9 th pillar (Autodesk Fusion 360 design; units mm, degrees)
description: Spur Gear; Module: 1.27; Num Teeth: 9; Pressure Angle: 20.0; Backlash: 0.00 mm
part number: 2026-06-06-19-48-23-059
Autodesk Fusion 360 part; units mm, degrees
sketch "Base Circle" plane through (0, 0, 0) normal (0, 0, 1) x (1, 0, 0)
  circle A0 centre (0, 0) radius 4.2456
  circle A1 centre (0, 0) radius 2.5
extrude "Extrude1" add sketch "Base Circle" along normal blind 1
sketch "Gear Tooth" plane through (0, 0, 0) normal (0, 0, 1) x (1, 0, 0)
  spline S0 degree 5 poles (5.2743, -1.0113) (5.279, -1.0122) (5.2884, -1.0138) (5.3026, -1.0158) (5.3217, -1.0174) (5.3456, -1.0181) (5.3698, -1.0179) (5.394, -1.0171) (5.4182, -1.016) (5.4425, -1.0146) (5.4668, -1.013) (5.4912, -1.0111) (5.5156, -1.0088) (5.5401, -1.0061) (5.5646, -1.0028) (5.5892, -0.9991) (5.6137, -0.995) (5.6383, -0.9906) (5.663, -0.9859) (5.6876, -0.981) (5.7122, -0.9757) (5.7369, -0.9702) (5.7616, -0.9644) (5.7863, -0.9583) (5.811, -0.9518) (5.8357, -0.9451) (5.8604, -0.9381) (5.8851, -0.9308) (5.9098, -0.9233) (5.9345, -0.9155) (5.9592, -0.9074) (5.9839, -0.8991) (6.0086, -0.8905) (6.0333, -0.8817) (6.058, -0.8726) (6.0827, -0.8632) (6.1073, -0.8537) (6.132, -0.8438) (6.1566, -0.8338) (6.1812, -0.8234) (6.2058, -0.8129) (6.2304, -0.8021) (6.255, -0.7911) (6.2795, -0.7799) (6.304, -0.7684) (6.3285, -0.7567) (6.353, -0.7448) (6.3774, -0.7326) (6.4018, -0.7203) (6.4262, -0.7077) (6.4505, -0.6948) (6.4748, -0.6818) (6.4991, -0.6686) (6.5233, -0.6551) (6.5475, -0.6414) (6.5717, -0.6275) (6.5958, -0.6134) (6.6199, -0.5991) (6.644, -0.5846) (6.668, -0.5698) (6.6919, -0.5549) (6.7159, -0.5397) (6.7397, -0.5244) (6.7636, -0.5088) (6.7874, -0.493) (6.8111, -0.4771) (6.8348, -0.4609) (6.8584, -0.4445) (6.882, -0.4279) (6.9055, -0.4112) (6.929, -0.3942) (6.9477, -0.3805) (6.9617, -0.3701) (6.9711, -0.3631) (6.9757, -0.3597) knots 0 0 0 0 0 0 0.01428571 0.02857143 0.04285714 0.05714286 0.07142857 0.08571429 0.1 0.11428571 0.12857143 0.14285714 0.15714286 0.17142857 0.18571429 0.2 0.21428571 0.22857143 0.24285714 0.25714286 0.27142857 0.28571429 0.3 0.31428571 0.32857143 0.34285714 0.35714286 0.37142857 0.38571429 0.4 0.41428571 0.42857143 0.44285714 0.45714286 0.47142857 0.48571429 0.5 0.51428571 0.52857143 0.54285714 0.55714286 0.57142857 0.58571429 0.6 0.61428571 0.62857143 0.64285714 0.65714286 0.67142857 0.68571429 0.7 0.71428571 0.72857143 0.74285714 0.75714286 0.77142857 0.78571429 0.8 0.81428571 0.82857143 0.84285714 0.85714286 0.87142857 0.88571429 0.9 0.91428571 0.92857143 0.94285714 0.95714286 0.97142857 0.98571429 1 1 1 1 1 1
  spline S1 degree 5 poles (5.2743, 1.0113) (5.279, 1.0122) (5.2884, 1.0138) (5.3026, 1.0158) (5.3217, 1.0174) (5.3456, 1.0181) (5.3698, 1.0179) (5.394, 1.0171) (5.4182, 1.016) (5.4425, 1.0146) (5.4668, 1.013) (5.4912, 1.0111) (5.5156, 1.0088) (5.5401, 1.0061) (5.5646, 1.0028) (5.5892, 0.9991) (5.6137, 0.995) (5.6383, 0.9906) (5.663, 0.9859) (5.6876, 0.981) (5.7122, 0.9757) (5.7369, 0.9702) (5.7616, 0.9644) (5.7863, 0.9583) (5.811, 0.9518) (5.8357, 0.9451) (5.8604, 0.9381) (5.8851, 0.9308) (5.9098, 0.9233) (5.9345, 0.9155) (5.9592, 0.9074) (5.9839, 0.8991) (6.0086, 0.8905) (6.0333, 0.8817) (6.058, 0.8726) (6.0827, 0.8632) (6.1073, 0.8537) (6.132, 0.8438) (6.1566, 0.8338) (6.1812, 0.8234) (6.2058, 0.8129) (6.2304, 0.8021) (6.255, 0.7911) (6.2795, 0.7799) (6.304, 0.7684) (6.3285, 0.7567) (6.353, 0.7448) (6.3774, 0.7326) (6.4018, 0.7203) (6.4262, 0.7077) (6.4505, 0.6948) (6.4748, 0.6818) (6.4991, 0.6686) (6.5233, 0.6551) (6.5475, 0.6414) (6.5717, 0.6275) (6.5958, 0.6134) (6.6199, 0.5991) (6.644, 0.5846) (6.668, 0.5698) (6.6919, 0.5549) (6.7159, 0.5397) (6.7397, 0.5244) (6.7636, 0.5088) (6.7874, 0.493) (6.8111, 0.4771) (6.8348, 0.4609) (6.8584, 0.4445) (6.882, 0.4279) (6.9055, 0.4112) (6.929, 0.3942) (6.9477, 0.3805) (6.9617, 0.3701) (6.9711, 0.3631) (6.9757, 0.3597) knots 0 0 0 0 0 0 0.01428571 0.02857143 0.04285714 0.05714286 0.07142857 0.08571429 0.1 0.11428571 0.12857143 0.14285714 0.15714286 0.17142857 0.18571429 0.2 0.21428571 0.22857143 0.24285714 0.25714286 0.27142857 0.28571429 0.3 0.31428571 0.32857143 0.34285714 0.35714286 0.37142857 0.38571429 0.4 0.41428571 0.42857143 0.44285714 0.45714286 0.47142857 0.48571429 0.5 0.51428571 0.52857143 0.54285714 0.55714286 0.57142857 0.58571429 0.6 0.61428571 0.62857143 0.64285714 0.65714286 0.67142857 0.68571429 0.7 0.71428571 0.72857143 0.74285714 0.75714286 0.77142857 0.78571429 0.8 0.81428571 0.82857143 0.84285714 0.85714286 0.87142857 0.88571429 0.9 0.91428571 0.92857143 0.94285714 0.95714286 0.97142857 0.98571429 1 1 1 1 1 1
  arc A0 (6.9757, -0.3597) -> (6.9757, 0.3597) centre (0, 0) ccw
  line L0 (4.1598, -0.7976) -> (5.2743, -1.0113)
  line L1 (4.1598, 0.7976) -> (5.2743, 1.0113)
  line L2 (4.1598, -0.7976) -> (4.1598, 0.7976)
  point P0 (5.3906, -1.0171)
  point P1 (5.5093, -1.0094)
  point P2 (5.6296, -0.9922)
  point P3 (5.751, -0.9669)
  point P4 (5.8732, -0.9343)
  point P5 (5.9959, -0.8949)
  point P6 (6.1191, -0.8489)
  point P7 (6.2424, -0.7967)
  point P8 (6.3656, -0.7384)
  point P9 (6.4887, -0.6742)
  point P10 (6.6115, -0.6041)
  point P11 (6.7336, -0.5282)
  point P12 (6.8551, -0.4467)
  point P13 (5.3906, 1.0171)
  point P14 (5.5093, 1.0094)
  point P15 (5.6296, 0.9922)
  point P16 (5.751, 0.9669)
  point P17 (5.8732, 0.9343)
  point P18 (5.9959, 0.8949)
  point P19 (6.1191, 0.8489)
  point P20 (6.2424, 0.7967)
  point P21 (6.3656, 0.7384)
  point P22 (6.4887, 0.6742)
  point P23 (6.6115, 0.6041)
  point P24 (6.7336, 0.5282)
  point P25 (6.8551, 0.4467)
extrude "Extrude2" add sketch "Gear Tooth" along normal blind 1
fillet "Fillet1" radius 0.2 2 edges at (4.1697, -0.7995, 0.5) (4.1697, 0.7995, 0.5)
pattern_circular "C-Pattern1" count 9 over 360 about axis through (0, 0, 0) along (0, 0, 1) of "Extrude2", "Fillet1"
sketch "Diametrial Pitch Circle" plane through (0, 0, 0) normal (0, 0, 1) x (1, 0, 0)
  circle A0 centre (0, 0) radius 5.715 construction
extrude "Extrude3" add 1 faces at (-1.8218, -3.1555, 1) along direction (0, 0, 1) blind 23
sketch "Sketch4" plane through (0, 0, 24) normal (0, 0, 1) x (1, 0, 0)
  arc A0 (3.7973, -1.8989) -> (4.1295, -0.9863) centre (0, 0) ccw
  arc A1 (4.3617, -0.8363) -> (4.1295, -0.9863) centre (4.324, -1.0327) ccw
  line L0 (4.3617, -0.8363) -> (5.2743, -1.0113)
  spline S0 degree 5 poles (5.2743, -1.0113) (5.279, -1.0122) (5.2884, -1.0138) (5.3026, -1.0158) (5.3217, -1.0174) (5.3456, -1.0181) (5.3698, -1.0179) (5.394, -1.0171) (5.4182, -1.016) (5.4425, -1.0146) (5.4668, -1.013) (5.4912, -1.0111) (5.5156, -1.0088) (5.5401, -1.0061) (5.5646, -1.0028) (5.5892, -0.9991) (5.6137, -0.995) (5.6383, -0.9906) (5.663, -0.9859) (5.6876, -0.981) (5.7122, -0.9757) (5.7369, -0.9702) (5.7616, -0.9644) (5.7863, -0.9583) (5.811, -0.9518) (5.8357, -0.9451) (5.8604, -0.9381) (5.8851, -0.9308) (5.9098, -0.9233) (5.9345, -0.9155) (5.9592, -0.9074) (5.9839, -0.8991) (6.0086, -0.8905) (6.0333, -0.8817) (6.058, -0.8726) (6.0827, -0.8632) (6.1073, -0.8537) (6.132, -0.8438) (6.1566, -0.8338) (6.1812, -0.8234) (6.2058, -0.8129) (6.2304, -0.8021) (6.255, -0.7911) (6.2795, -0.7799) (6.304, -0.7684) (6.3285, -0.7567) (6.353, -0.7448) (6.3774, -0.7326) (6.4018, -0.7203) (6.4262, -0.7077) (6.4505, -0.6948) (6.4748, -0.6818) (6.4991, -0.6686) (6.5233, -0.6551) (6.5475, -0.6414) (6.5717, -0.6275) (6.5958, -0.6134) (6.6199, -0.5991) (6.644, -0.5846) (6.668, -0.5698) (6.6919, -0.5549) (6.7159, -0.5397) (6.7397, -0.5244) (6.7636, -0.5088) (6.7874, -0.493) (6.8111, -0.4771) (6.8348, -0.4609) (6.8584, -0.4445) (6.882, -0.4279) (6.9055, -0.4112) (6.929, -0.3942) (6.9477, -0.3805) (6.9617, -0.3701) (6.9711, -0.3631) (6.9757, -0.3597) knots 0 0 0 0 0 0 0.01428571 0.02857143 0.04285714 0.05714286 0.07142857 0.08571429 0.1 0.11428571 0.12857143 0.14285714 0.15714286 0.17142857 0.18571429 0.2 0.21428571 0.22857143 0.24285714 0.25714286 0.27142857 0.28571429 0.3 0.31428571 0.32857143 0.34285714 0.35714286 0.37142857 0.38571429 0.4 0.41428571 0.42857143 0.44285714 0.45714286 0.47142857 0.48571429 0.5 0.51428571 0.52857143 0.54285714 0.55714286 0.57142857 0.58571429 0.6 0.61428571 0.62857143 0.64285714 0.65714286 0.67142857 0.68571429 0.7 0.71428571 0.72857143 0.74285714 0.75714286 0.77142857 0.78571429 0.8 0.81428571 0.82857143 0.84285714 0.85714286 0.87142857 0.88571429 0.9 0.91428571 0.92857143 0.94285714 0.95714286 0.97142857 0.98571429 1 1 1 1 1 1
  arc A2 (6.9757, -0.3597) -> (6.9757, 0.3597) centre (0, 0) ccw
  spline S1 degree 5 poles (6.9757, 0.3597) (6.9711, 0.3631) (6.9617, 0.3701) (6.9477, 0.3805) (6.929, 0.3942) (6.9055, 0.4112) (6.882, 0.4279) (6.8584, 0.4445) (6.8348, 0.4609) (6.8111, 0.4771) (6.7874, 0.493) (6.7636, 0.5088) (6.7397, 0.5244) (6.7159, 0.5397) (6.6919, 0.5549) (6.668, 0.5698) (6.644, 0.5846) (6.6199, 0.5991) (6.5958, 0.6134) (6.5717, 0.6275) (6.5475, 0.6414) (6.5233, 0.6551) (6.4991, 0.6686) (6.4748, 0.6818) (6.4505, 0.6948) (6.4262, 0.7077) (6.4018, 0.7203) (6.3774, 0.7326) (6.353, 0.7448) (6.3285, 0.7567) (6.304, 0.7684) (6.2795, 0.7799) (6.255, 0.7911) (6.2304, 0.8021) (6.2058, 0.8129) (6.1812, 0.8234) (6.1566, 0.8338) (6.132, 0.8438) (6.1073, 0.8537) (6.0827, 0.8632) (6.058, 0.8726) (6.0333, 0.8817) (6.0086, 0.8905) (5.9839, 0.8991) (5.9592, 0.9074) (5.9345, 0.9155) (5.9098, 0.9233) (5.8851, 0.9308) (5.8604, 0.9381) (5.8357, 0.9451) (5.811, 0.9518) (5.7863, 0.9583) (5.7616, 0.9644) (5.7369, 0.9702) (5.7122, 0.9757) (5.6876, 0.981) (5.663, 0.9859) (5.6383, 0.9906) (5.6137, 0.995) (5.5892, 0.9991) (5.5646, 1.0028) (5.5401, 1.0061) (5.5156, 1.0088) (5.4912, 1.0111) (5.4668, 1.013) (5.4425, 1.0146) (5.4182, 1.016) (5.394, 1.0171) (5.3698, 1.0179) (5.3456, 1.0181) (5.3217, 1.0174) (5.3026, 1.0158) (5.2884, 1.0138) (5.279, 1.0122) (5.2743, 1.0113) knots -1 -1 -1 -1 -1 -1 -0.98571429 -0.97142857 -0.95714286 -0.94285714 -0.92857143 -0.91428571 -0.9 -0.88571429 -0.87142857 -0.85714286 -0.84285714 -0.82857143 -0.81428571 -0.8 -0.78571429 -0.77142857 -0.75714286 -0.74285714 -0.72857143 -0.71428571 -0.7 -0.68571429 -0.67142857 -0.65714286 -0.64285714 -0.62857143 -0.61428571 -0.6 -0.58571429 -0.57142857 -0.55714286 -0.54285714 -0.52857143 -0.51428571 -0.5 -0.48571429 -0.47142857 -0.45714286 -0.44285714 -0.42857143 -0.41428571 -0.4 -0.38571429 -0.37142857 -0.35714286 -0.34285714 -0.32857143 -0.31428571 -0.3 -0.28571429 -0.27142857 -0.25714286 -0.24285714 -0.22857143 -0.21428571 -0.2 -0.18571429 -0.17142857 -0.15714286 -0.14285714 -0.12857143 -0.11428571 -0.1 -0.08571429 -0.07142857 -0.05714286 -0.04285714 -0.02857143 -0.01428571 0 0 0 0 0 0
  line L1 (5.2743, 1.0113) -> (4.3617, 0.8363)
  arc A3 (4.1295, 0.9863) -> (4.3617, 0.8363) centre (4.324, 1.0327) ccw
  arc A4 (4.1295, 0.9863) -> (3.7973, 1.8989) centre (0, 0) ccw
  arc A5 (3.8788, 2.163) -> (3.7973, 1.8989) centre (3.9762, 1.9883) ccw
  line L2 (3.8788, 2.163) -> (4.6904, 2.6156)
  spline S2 degree 5 poles (4.6904, 2.6156) (4.6945, 2.6179) (4.7028, 2.6227) (4.7149, 2.6303) (4.7306, 2.6413) (4.7494, 2.6562) (4.7678, 2.6719) (4.7858, 2.688) (4.8036, 2.7045) (4.8214, 2.7211) (4.839, 2.738) (4.8565, 2.7551) (4.8737, 2.7726) (4.8906, 2.7904) (4.9073, 2.8087) (4.9238, 2.8273) (4.94, 2.8462) (4.956, 2.8654) (4.9718, 2.8848) (4.9875, 2.9044) (5.003, 2.9243) (5.0184, 2.9444) (5.0335, 2.9647) (5.0485, 2.9853) (5.0633, 3.0061) (5.0779, 3.0271) (5.0923, 3.0484) (5.1066, 3.0698) (5.1206, 3.0915) (5.1346, 3.1134) (5.1483, 3.1354) (5.1619, 3.1577) (5.1753, 3.1801) (5.1885, 3.2028) (5.2016, 3.2256) (5.2145, 3.2486) (5.2272, 3.2718) (5.2398, 3.2952) (5.2522, 3.3187) (5.2644, 3.3424) (5.2765, 3.3663) (5.2884, 3.3904) (5.3001, 3.4146) (5.3117, 3.439) (5.3231, 3.4635) (5.3343, 3.4882) (5.3454, 3.5131) (5.3563, 3.5381) (5.367, 3.5632) (5.3776, 3.5886) (5.388, 3.614) (5.3983, 3.6396) (5.4083, 3.6654) (5.4182, 3.6913) (5.428, 3.7173) (5.4376, 3.7435) (5.447, 3.7698) (5.4562, 3.7963) (5.4653, 3.8229) (5.4742, 3.8496) (5.483, 3.8764) (5.4916, 3.9034) (5.5, 3.9305) (5.5082, 3.9578) (5.5163, 3.9851) (5.5242, 4.0126) (5.532, 4.0402) (5.5396, 4.068) (5.547, 4.0958) (5.5542, 4.1238) (5.5613, 4.1519) (5.5668, 4.1744) (5.5709, 4.1914) (5.5736, 4.2027) (5.5749, 4.2084) knots 0 0 0 0 0 0 0.01428571 0.02857143 0.04285714 0.05714286 0.07142857 0.08571429 0.1 0.11428571 0.12857143 0.14285714 0.15714286 0.17142857 0.18571429 0.2 0.21428571 0.22857143 0.24285714 0.25714286 0.27142857 0.28571429 0.3 0.31428571 0.32857143 0.34285714 0.35714286 0.37142857 0.38571429 0.4 0.41428571 0.42857143 0.44285714 0.45714286 0.47142857 0.48571429 0.5 0.51428571 0.52857143 0.54285714 0.55714286 0.57142857 0.58571429 0.6 0.61428571 0.62857143 0.64285714 0.65714286 0.67142857 0.68571429 0.7 0.71428571 0.72857143 0.74285714 0.75714286 0.77142857 0.78571429 0.8 0.81428571 0.82857143 0.84285714 0.85714286 0.87142857 0.88571429 0.9 0.91428571 0.92857143 0.94285714 0.95714286 0.97142857 0.98571429 1 1 1 1 1 1
  arc A6 (5.5749, 4.2084) -> (5.1125, 4.7594) centre (0, 0) ccw
  spline S3 degree 5 poles (5.1125, 4.7594) (5.1067, 4.7591) (5.0951, 4.7584) (5.0777, 4.7574) (5.0545, 4.7558) (5.0256, 4.7538) (4.9968, 4.7515) (4.9681, 4.749) (4.9395, 4.7464) (4.9109, 4.7435) (4.8825, 4.7405) (4.8542, 4.7373) (4.8259, 4.7339) (4.7977, 4.7303) (4.7697, 4.7266) (4.7417, 4.7226) (4.7138, 4.7185) (4.6861, 4.7141) (4.6584, 4.7096) (4.6309, 4.7049) (4.6034, 4.7) (4.5761, 4.6949) (4.5489, 4.6897) (4.5217, 4.6842) (4.4947, 4.6786) (4.4679, 4.6728) (4.4411, 4.6667) (4.4144, 4.6605) (4.3879, 4.6541) (4.3615, 4.6475) (4.3352, 4.6408) (4.3091, 4.6338) (4.2831, 4.6266) (4.2572, 4.6193) (4.2314, 4.6118) (4.2058, 4.604) (4.1803, 4.5961) (4.155, 4.588) (4.1298, 4.5797) (4.1047, 4.5712) (4.0798, 4.5624) (4.0551, 4.5535) (4.0305, 4.5444) (4.0061, 4.5351) (3.9818, 4.5256) (3.9577, 4.5159) (3.9337, 4.506) (3.9099, 4.4959) (3.8863, 4.4856) (3.8629, 4.4751) (3.8396, 4.4644) (3.8166, 4.4534) (3.7937, 4.4423) (3.7711, 4.4309) (3.7486, 4.4192) (3.7264, 4.4074) (3.7043, 4.3953) (3.6825, 4.3831) (3.6608, 4.3707) (3.6393, 4.358) (3.6181, 4.3451) (3.5973, 4.3318) (3.5768, 4.3182) (3.5566, 4.3043) (3.5367, 4.2901) (3.517, 4.2756) (3.4975, 4.261) (3.4782, 4.2463) (3.4592, 4.2314) (3.4406, 4.216) (3.4227, 4.2001) (3.4091, 4.1866) (3.3995, 4.1759) (3.3933, 4.1686) (3.3903, 4.1649) knots -1 -1 -1 -1 -1 -1 -0.98571429 -0.97142857 -0.95714286 -0.94285714 -0.92857143 -0.91428571 -0.9 -0.88571429 -0.87142857 -0.85714286 -0.84285714 -0.82857143 -0.81428571 -0.8 -0.78571429 -0.77142857 -0.75714286 -0.74285714 -0.72857143 -0.71428571 -0.7 -0.68571429 -0.67142857 -0.65714286 -0.64285714 -0.62857143 -0.61428571 -0.6 -0.58571429 -0.57142857 -0.55714286 -0.54285714 -0.52857143 -0.51428571 -0.5 -0.48571429 -0.47142857 -0.45714286 -0.44285714 -0.42857143 -0.41428571 -0.4 -0.38571429 -0.37142857 -0.35714286 -0.34285714 -0.32857143 -0.31428571 -0.3 -0.28571429 -0.27142857 -0.25714286 -0.24285714 -0.22857143 -0.21428571 -0.2 -0.18571429 -0.17142857 -0.15714286 -0.14285714 -0.12857143 -0.11428571 -0.1 -0.08571429 -0.07142857 -0.05714286 -0.04285714 -0.02857143 -0.01428571 0 0 0 0 0 0
  line L3 (3.3903, 4.1649) -> (2.8037, 3.4443)
  arc A7 (2.5294, 3.4099) -> (2.8037, 3.4443) centre (2.6486, 3.5705) ccw
  arc A8 (2.5294, 3.4099) -> (1.6883, 3.8955) centre (0, 0) ccw
  arc A9 (1.581, 4.1502) -> (1.6883, 3.8955) centre (1.7679, 4.079) ccw
  line L4 (1.581, 4.1502) -> (1.9118, 5.0185)
  spline S4 degree 5 poles (1.9118, 5.0185) (1.9135, 5.023) (1.9167, 5.032) (1.9211, 5.0457) (1.926, 5.0641) (1.9309, 5.0876) (1.9349, 5.1114) (1.9383, 5.1354) (1.9414, 5.1595) (1.9443, 5.1836) (1.947, 5.2079) (1.9493, 5.2322) (1.9513, 5.2567) (1.9528, 5.2812) (1.9539, 5.3059) (1.9545, 5.3308) (1.9547, 5.3557) (1.9547, 5.3807) (1.9543, 5.4057) (1.9537, 5.4308) (1.9528, 5.456) (1.9517, 5.4813) (1.9502, 5.5066) (1.9485, 5.532) (1.9464, 5.5574) (1.9441, 5.5829) (1.9415, 5.6085) (1.9386, 5.6341) (1.9355, 5.6597) (1.9321, 5.6854) (1.9284, 5.7111) (1.9245, 5.7369) (1.9204, 5.7627) (1.9159, 5.7886) (1.9113, 5.8145) (1.9064, 5.8404) (1.9012, 5.8663) (1.8958, 5.8923) (1.8902, 5.9183) (1.8843, 5.9443) (1.8782, 5.9704) (1.8718, 5.9965) (1.8653, 6.0226) (1.8585, 6.0487) (1.8514, 6.0748) (1.8441, 6.1009) (1.8366, 6.1271) (1.8289, 6.1533) (1.821, 6.1795) (1.8128, 6.2057) (1.8044, 6.2318) (1.7958, 6.2581) (1.787, 6.2843) (1.7779, 6.3105) (1.7686, 6.3367) (1.7591, 6.3629) (1.7494, 6.3891) (1.7395, 6.4153) (1.7294, 6.4415) (1.719, 6.4677) (1.7085, 6.4939) (1.6977, 6.5201) (1.6867, 6.5463) (1.6755, 6.5725) (1.6641, 6.5986) (1.6525, 6.6248) (1.6407, 6.6509) (1.6287, 6.677) (1.6165, 6.7031) (1.6041, 6.7292) (1.5914, 6.7552) (1.5812, 6.7761) (1.5734, 6.7917) (1.5681, 6.8021) (1.5655, 6.8073) knots 0 0 0 0 0 0 0.01428571 0.02857143 0.04285714 0.05714286 0.07142857 0.08571429 0.1 0.11428571 0.12857143 0.14285714 0.15714286 0.17142857 0.18571429 0.2 0.21428571 0.22857143 0.24285714 0.25714286 0.27142857 0.28571429 0.3 0.31428571 0.32857143 0.34285714 0.35714286 0.37142857 0.38571429 0.4 0.41428571 0.42857143 0.44285714 0.45714286 0.47142857 0.48571429 0.5 0.51428571 0.52857143 0.54285714 0.55714286 0.57142857 0.58571429 0.6 0.61428571 0.62857143 0.64285714 0.65714286 0.67142857 0.68571429 0.7 0.71428571 0.72857143 0.74285714 0.75714286 0.77142857 0.78571429 0.8 0.81428571 0.82857143 0.84285714 0.85714286 0.87142857 0.88571429 0.9 0.91428571 0.92857143 0.94285714 0.95714286 0.97142857 0.98571429 1 1 1 1 1 1
  arc A10 (1.5655, 6.8073) -> (0.8571, 6.9322) centre (0, 0) ccw
  spline S5 degree 5 poles (0.8571, 6.9322) (0.8529, 6.9282) (0.8444, 6.9202) (0.8317, 6.9082) (0.815, 6.8922) (0.7942, 6.872) (0.7736, 6.8517) (0.7532, 6.8314) (0.733, 6.811) (0.7129, 6.7904) (0.6931, 6.7698) (0.6734, 6.7492) (0.654, 6.7284) (0.6347, 6.7076) (0.6156, 6.6866) (0.5967, 6.6656) (0.578, 6.6445) (0.5596, 6.6234) (0.5413, 6.6021) (0.5232, 6.5808) (0.5053, 6.5594) (0.4876, 6.538) (0.4702, 6.5164) (0.4529, 6.4948) (0.4358, 6.4732) (0.419, 6.4514) (0.4023, 6.4296) (0.3859, 6.4077) (0.3697, 6.3858) (0.3537, 6.3638) (0.3379, 6.3417) (0.3224, 6.3195) (0.3071, 6.2973) (0.292, 6.275) (0.2771, 6.2527) (0.2624, 6.2303) (0.248, 6.2079) (0.2338, 6.1854) (0.2198, 6.1628) (0.2061, 6.1402) (0.1926, 6.1175) (0.1794, 6.0948) (0.1664, 6.072) (0.1537, 6.0492) (0.1412, 6.0263) (0.129, 6.0033) (0.117, 5.9804) (0.1053, 5.9573) (0.0938, 5.9343) (0.0826, 5.9111) (0.0717, 5.888) (0.0611, 5.8648) (0.0507, 5.8415) (0.0407, 5.8182) (0.031, 5.7949) (0.0216, 5.7715) (0.0124, 5.7481) (0.0035, 5.7247) (-0.0051, 5.7012) (-0.0134, 5.6777) (-0.0213, 5.6542) (-0.0288, 5.6306) (-0.0357, 5.607) (-0.0422, 5.5834) (-0.0483, 5.5597) (-0.0541, 5.536) (-0.0597, 5.5123) (-0.065, 5.4886) (-0.07, 5.4649) (-0.0744, 5.4412) (-0.0778, 5.4175) (-0.0795, 5.3984) (-0.0801, 5.3841) (-0.0801, 5.3745) (-0.08, 5.3697) knots -1 -1 -1 -1 -1 -1 -0.98571429 -0.97142857 -0.95714286 -0.94285714 -0.92857143 -0.91428571 -0.9 -0.88571429 -0.87142857 -0.85714286 -0.84285714 -0.82857143 -0.81428571 -0.8 -0.78571429 -0.77142857 -0.75714286 -0.74285714 -0.72857143 -0.71428571 -0.7 -0.68571429 -0.67142857 -0.65714286 -0.64285714 -0.62857143 -0.61428571 -0.6 -0.58571429 -0.57142857 -0.55714286 -0.54285714 -0.52857143 -0.51428571 -0.5 -0.48571429 -0.47142857 -0.45714286 -0.44285714 -0.42857143 -0.41428571 -0.4 -0.38571429 -0.37142857 -0.35714286 -0.34285714 -0.32857143 -0.31428571 -0.3 -0.28571429 -0.27142857 -0.25714286 -0.24285714 -0.22857143 -0.21428571 -0.2 -0.18571429 -0.17142857 -0.15714286 -0.14285714 -0.12857143 -0.11428571 -0.1 -0.08571429 -0.07142857 -0.05714286 -0.04285714 -0.02857143 -0.01428571 0 0 0 0 0 0
  line L5 (-0.08, 5.3697) -> (-0.0662, 4.4406)
  arc A11 (-0.2542, 4.238) -> (-0.0662, 4.4406) centre (-0.2662, 4.4376) ccw
  arc A12 (-0.2542, 4.238) -> (-1.2106, 4.0694) centre (0, 0) ccw
  arc A13 (-1.4566, 4.1955) -> (-1.2106, 4.0694) centre (-1.2676, 4.261) ccw
  line L6 (-1.4566, 4.1955) -> (-1.7613, 5.0733)
  spline S6 degree 5 poles (-1.7613, 5.0733) (-1.7629, 5.0778) (-1.7662, 5.0868) (-1.7716, 5.1001) (-1.7797, 5.1174) (-1.7911, 5.1385) (-1.8033, 5.1593) (-1.8161, 5.1799) (-1.8292, 5.2003) (-1.8426, 5.2207) (-1.8561, 5.2409) (-1.8699, 5.2611) (-1.8841, 5.2811) (-1.8988, 5.3009) (-1.9138, 5.3205) (-1.9293, 5.3399) (-1.9451, 5.3591) (-1.9613, 5.3783) (-1.9776, 5.3972) (-1.9942, 5.4161) (-2.0111, 5.4348) (-2.0282, 5.4534) (-2.0456, 5.4719) (-2.0632, 5.4902) (-2.0812, 5.5084) (-2.0994, 5.5264) (-2.1178, 5.5443) (-2.1365, 5.5621) (-2.1553, 5.5797) (-2.1745, 5.5972) (-2.1938, 5.6145) (-2.2134, 5.6318) (-2.2331, 5.6489) (-2.2531, 5.6659) (-2.2733, 5.6827) (-2.2938, 5.6994) (-2.3144, 5.7159) (-2.3352, 5.7324) (-2.3563, 5.7487) (-2.3775, 5.7648) (-2.3989, 5.7809) (-2.4205, 5.7968) (-2.4424, 5.8125) (-2.4644, 5.8281) (-2.4865, 5.8436) (-2.5089, 5.859) (-2.5315, 5.8742) (-2.5542, 5.8893) (-2.5771, 5.9042) (-2.6002, 5.9191) (-2.6235, 5.9337) (-2.6469, 5.9483) (-2.6706, 5.9627) (-2.6943, 5.9769) (-2.7183, 5.991) (-2.7424, 6.005) (-2.7667, 6.0189) (-2.7911, 6.0326) (-2.8158, 6.0461) (-2.8405, 6.0595) (-2.8654, 6.0728) (-2.8905, 6.086) (-2.9158, 6.099) (-2.9412, 6.1118) (-2.9667, 6.1245) (-2.9924, 6.1371) (-3.0182, 6.1495) (-3.0442, 6.1618) (-3.0704, 6.1739) (-3.0967, 6.1859) (-3.1231, 6.1978) (-3.1443, 6.2071) (-3.1603, 6.2141) (-3.171, 6.2187) (-3.1764, 6.221) knots 0 0 0 0 0 0 0.01428571 0.02857143 0.04285714 0.05714286 0.07142857 0.08571429 0.1 0.11428571 0.12857143 0.14285714 0.15714286 0.17142857 0.18571429 0.2 0.21428571 0.22857143 0.24285714 0.25714286 0.27142857 0.28571429 0.3 0.31428571 0.32857143 0.34285714 0.35714286 0.37142857 0.38571429 0.4 0.41428571 0.42857143 0.44285714 0.45714286 0.47142857 0.48571429 0.5 0.51428571 0.52857143 0.54285714 0.55714286 0.57142857 0.58571429 0.6 0.61428571 0.62857143 0.64285714 0.65714286 0.67142857 0.68571429 0.7 0.71428571 0.72857143 0.74285714 0.75714286 0.77142857 0.78571429 0.8 0.81428571 0.82857143 0.84285714 0.85714286 0.87142857 0.88571429 0.9 0.91428571 0.92857143 0.94285714 0.95714286 0.97142857 0.98571429 1 1 1 1 1 1
  arc A14 (-3.1764, 6.221) -> (-3.7993, 5.8613) centre (0, 0) ccw
  spline S7 degree 5 poles (-3.7993, 5.8613) (-3.8, 5.8556) (-3.8014, 5.844) (-3.8034, 5.8266) (-3.8059, 5.8036) (-3.8088, 5.7747) (-3.8116, 5.746) (-3.8142, 5.7173) (-3.8165, 5.6886) (-3.8187, 5.66) (-3.8206, 5.6315) (-3.8224, 5.603) (-3.824, 5.5746) (-3.8253, 5.5463) (-3.8265, 5.518) (-3.8275, 5.4897) (-3.8282, 5.4616) (-3.8288, 5.4335) (-3.8291, 5.4055) (-3.8293, 5.3775) (-3.8292, 5.3496) (-3.829, 5.3218) (-3.8285, 5.2941) (-3.8279, 5.2664) (-3.827, 5.2389) (-3.8259, 5.2114) (-3.8247, 5.184) (-3.8232, 5.1567) (-3.8215, 5.1294) (-3.8196, 5.1023) (-3.8175, 5.0752) (-3.8151, 5.0483) (-3.8126, 5.0214) (-3.8099, 4.9946) (-3.8069, 4.968) (-3.8037, 4.9414) (-3.8004, 4.9149) (-3.7968, 4.8885) (-3.793, 4.8623) (-3.7889, 4.8361) (-3.7847, 4.8101) (-3.7802, 4.7842) (-3.7755, 4.7584) (-3.7706, 4.7327) (-3.7654, 4.7072) (-3.7601, 4.6817) (-3.7545, 4.6564) (-3.7487, 4.6312) (-3.7426, 4.6062) (-3.7363, 4.5813) (-3.7298, 4.5565) (-3.723, 4.5319) (-3.716, 4.5075) (-3.7087, 4.4832) (-3.7011, 4.4591) (-3.6933, 4.4351) (-3.6853, 4.4113) (-3.6771, 4.3876) (-3.6686, 4.3641) (-3.6598, 4.3408) (-3.6508, 4.3177) (-3.6413, 4.2948) (-3.6315, 4.2723) (-3.6213, 4.25) (-3.6107, 4.2279) (-3.5999, 4.206) (-3.589, 4.1843) (-3.5778, 4.1628) (-3.5664, 4.1414) (-3.5545, 4.1204) (-3.5419, 4.1) (-3.531, 4.0843) (-3.5222, 4.073) (-3.5161, 4.0656) (-3.5129, 4.062) knots -1 -1 -1 -1 -1 -1 -0.98571429 -0.97142857 -0.95714286 -0.94285714 -0.92857143 -0.91428571 -0.9 -0.88571429 -0.87142857 -0.85714286 -0.84285714 -0.82857143 -0.81428571 -0.8 -0.78571429 -0.77142857 -0.75714286 -0.74285714 -0.72857143 -0.71428571 -0.7 -0.68571429 -0.67142857 -0.65714286 -0.64285714 -0.62857143 -0.61428571 -0.6 -0.58571429 -0.57142857 -0.55714286 -0.54285714 -0.52857143 -0.51428571 -0.5 -0.48571429 -0.47142857 -0.45714286 -0.44285714 -0.42857143 -0.41428571 -0.4 -0.38571429 -0.37142857 -0.35714286 -0.34285714 -0.32857143 -0.31428571 -0.3 -0.28571429 -0.27142857 -0.25714286 -0.24285714 -0.22857143 -0.21428571 -0.2 -0.18571429 -0.17142857 -0.15714286 -0.14285714 -0.12857143 -0.11428571 -0.1 -0.08571429 -0.07142857 -0.05714286 -0.04285714 -0.02857143 -0.01428571 0 0 0 0 0 0
  line L7 (-3.5129, 4.062) -> (-2.9051, 3.3592)
  arc A15 (-2.9189, 3.0831) -> (-2.9051, 3.3592) centre (-3.0564, 3.2283) ccw
  arc A16 (-2.9189, 3.0831) -> (-3.5431, 2.3391) centre (0, 0) ccw
  arc A17 (-3.8126, 2.2776) -> (-3.5431, 2.3391) centre (-3.71, 2.4493) ccw
  line L8 (-3.8126, 2.2776) -> (-4.6103, 2.7542)
  spline S8 degree 5 poles (-4.6103, 2.7542) (-4.6144, 2.7566) (-4.6227, 2.7614) (-4.6354, 2.7681) (-4.6528, 2.7761) (-4.675, 2.785) (-4.6978, 2.7931) (-4.7208, 2.8006) (-4.744, 2.8078) (-4.7673, 2.8149) (-4.7907, 2.8217) (-4.8142, 2.8283) (-4.838, 2.8345) (-4.8619, 2.8402) (-4.886, 2.8455) (-4.9104, 2.8505) (-4.9349, 2.855) (-4.9595, 2.8593) (-4.9842, 2.8633) (-5.0091, 2.8671) (-5.034, 2.8706) (-5.0591, 2.8739) (-5.0843, 2.8768) (-5.1096, 2.8795) (-5.135, 2.8819) (-5.1605, 2.884) (-5.1861, 2.8859) (-5.2118, 2.8875) (-5.2376, 2.8889) (-5.2635, 2.89) (-5.2895, 2.8908) (-5.3156, 2.8915) (-5.3417, 2.8919) (-5.3679, 2.892) (-5.3942, 2.8919) (-5.4206, 2.8916) (-5.4471, 2.891) (-5.4736, 2.8902) (-5.5002, 2.8892) (-5.5268, 2.8879) (-5.5535, 2.8864) (-5.5803, 2.8847) (-5.6072, 2.8827) (-5.6341, 2.8806) (-5.661, 2.8782) (-5.688, 2.8755) (-5.7151, 2.8727) (-5.7422, 2.8696) (-5.7694, 2.8664) (-5.7966, 2.8629) (-5.8238, 2.8591) (-5.8511, 2.8552) (-5.8785, 2.8511) (-5.9059, 2.8467) (-5.9333, 2.8421) (-5.9608, 2.8373) (-5.9883, 2.8323) (-6.0158, 2.8271) (-6.0434, 2.8217) (-6.071, 2.816) (-6.0986, 2.8102) (-6.1263, 2.8041) (-6.1539, 2.7979) (-6.1817, 2.7914) (-6.2094, 2.7847) (-6.2372, 2.7778) (-6.2649, 2.7707) (-6.2927, 2.7634) (-6.3206, 2.7559) (-6.3484, 2.7482) (-6.3763, 2.7403) (-6.3986, 2.7338) (-6.4153, 2.7288) (-6.4265, 2.7255) (-6.432, 2.7238) knots 0 0 0 0 0 0 0.01428571 0.02857143 0.04285714 0.05714286 0.07142857 0.08571429 0.1 0.11428571 0.12857143 0.14285714 0.15714286 0.17142857 0.18571429 0.2 0.21428571 0.22857143 0.24285714 0.25714286 0.27142857 0.28571429 0.3 0.31428571 0.32857143 0.34285714 0.35714286 0.37142857 0.38571429 0.4 0.41428571 0.42857143 0.44285714 0.45714286 0.47142857 0.48571429 0.5 0.51428571 0.52857143 0.54285714 0.55714286 0.57142857 0.58571429 0.6 0.61428571 0.62857143 0.64285714 0.65714286 0.67142857 0.68571429 0.7 0.71428571 0.72857143 0.74285714 0.75714286 0.77142857 0.78571429 0.8 0.81428571 0.82857143 0.84285714 0.85714286 0.87142857 0.88571429 0.9 0.91428571 0.92857143 0.94285714 0.95714286 0.97142857 0.98571429 1 1 1 1 1 1
  arc A18 (-6.432, 2.7238) -> (-6.6781, 2.0479) centre (0, 0) ccw
  spline S9 degree 5 poles (-6.6781, 2.0479) (-6.6749, 2.043) (-6.6685, 2.0333) (-6.6588, 2.0187) (-6.6459, 1.9994) (-6.6297, 1.9754) (-6.6133, 1.9516) (-6.5968, 1.928) (-6.5802, 1.9045) (-6.5635, 1.8812) (-6.5466, 1.8581) (-6.5297, 1.8352) (-6.5126, 1.8124) (-6.4954, 1.7898) (-6.4781, 1.7674) (-6.4607, 1.7451) (-6.4432, 1.7231) (-6.4256, 1.7012) (-6.4079, 1.6795) (-6.39, 1.658) (-6.372, 1.6367) (-6.354, 1.6155) (-6.3358, 1.5946) (-6.3175, 1.5738) (-6.2991, 1.5533) (-6.2807, 1.5329) (-6.2621, 1.5127) (-6.2434, 1.4927) (-6.2246, 1.473) (-6.2056, 1.4534) (-6.1866, 1.434) (-6.1675, 1.4149) (-6.1483, 1.3959) (-6.129, 1.3772) (-6.1096, 1.3586) (-6.0901, 1.3403) (-6.0705, 1.3222) (-6.0508, 1.3043) (-6.031, 1.2867) (-6.0111, 1.2692) (-5.9911, 1.252) (-5.971, 1.235) (-5.9508, 1.2183) (-5.9306, 1.2018) (-5.9102, 1.1855) (-5.8897, 1.1695) (-5.8692, 1.1537) (-5.8485, 1.1382) (-5.8278, 1.1229) (-5.807, 1.1078) (-5.7861, 1.093) (-5.7651, 1.0785) (-5.744, 1.0643) (-5.7228, 1.0504) (-5.7015, 1.0368) (-5.6801, 1.0235) (-5.6586, 1.0104) (-5.6371, 0.9975) (-5.6155, 0.985) (-5.5938, 0.9727) (-5.572, 0.9609) (-5.5501, 0.9494) (-5.528, 0.9385) (-5.5059, 0.9279) (-5.4836, 0.9178) (-5.4613, 0.908) (-5.4389, 0.8984) (-5.4165, 0.8891) (-5.3941, 0.88) (-5.3715, 0.8716) (-5.3487, 0.8641) (-5.3302, 0.8591) (-5.3162, 0.8561) (-5.3068, 0.8544) (-5.3021, 0.8536) knots -1 -1 -1 -1 -1 -1 -0.98571429 -0.97142857 -0.95714286 -0.94285714 -0.92857143 -0.91428571 -0.9 -0.88571429 -0.87142857 -0.85714286 -0.84285714 -0.82857143 -0.81428571 -0.8 -0.78571429 -0.77142857 -0.75714286 -0.74285714 -0.72857143 -0.71428571 -0.7 -0.68571429 -0.67142857 -0.65714286 -0.64285714 -0.62857143 -0.61428571 -0.6 -0.58571429 -0.57142857 -0.55714286 -0.54285714 -0.52857143 -0.51428571 -0.5 -0.48571429 -0.47142857 -0.45714286 -0.44285714 -0.42857143 -0.41428571 -0.4 -0.38571429 -0.37142857 -0.35714286 -0.34285714 -0.32857143 -0.31428571 -0.3 -0.28571429 -0.27142857 -0.25714286 -0.24285714 -0.22857143 -0.21428571 -0.2 -0.18571429 -0.17142857 -0.15714286 -0.14285714 -0.12857143 -0.11428571 -0.1 -0.08571429 -0.07142857 -0.05714286 -0.04285714 -0.02857143 -0.01428571 0 0 0 0 0 0
  line L9 (-5.3021, 0.8536) -> (-4.3846, 0.7059)
  arc A19 (-4.2177, 0.4856) -> (-4.3846, 0.7059) centre (-4.4164, 0.5085) ccw
  arc A20 (-4.2177, 0.4856) -> (-4.2177, -0.4856) centre (0, 0) ccw
  arc A21 (-4.3846, -0.7059) -> (-4.2177, -0.4856) centre (-4.4164, -0.5085) ccw
  line L10 (-4.3846, -0.7059) -> (-5.3021, -0.8536)
  spline S10 degree 5 poles (-5.3021, -0.8536) (-5.3068, -0.8544) (-5.3162, -0.8561) (-5.3302, -0.8591) (-5.3487, -0.8641) (-5.3715, -0.8716) (-5.3941, -0.88) (-5.4165, -0.8891) (-5.4389, -0.8984) (-5.4613, -0.908) (-5.4836, -0.9178) (-5.5059, -0.9279) (-5.528, -0.9385) (-5.5501, -0.9494) (-5.572, -0.9609) (-5.5938, -0.9727) (-5.6155, -0.985) (-5.6371, -0.9975) (-5.6586, -1.0104) (-5.6801, -1.0235) (-5.7015, -1.0368) (-5.7228, -1.0504) (-5.744, -1.0643) (-5.7651, -1.0785) (-5.7861, -1.093) (-5.807, -1.1078) (-5.8278, -1.1229) (-5.8485, -1.1382) (-5.8692, -1.1537) (-5.8897, -1.1695) (-5.9102, -1.1855) (-5.9306, -1.2018) (-5.9508, -1.2183) (-5.971, -1.235) (-5.9911, -1.252) (-6.0111, -1.2692) (-6.031, -1.2867) (-6.0508, -1.3043) (-6.0705, -1.3222) (-6.0901, -1.3403) (-6.1096, -1.3586) (-6.129, -1.3772) (-6.1483, -1.3959) (-6.1675, -1.4149) (-6.1866, -1.434) (-6.2056, -1.4534) (-6.2246, -1.473) (-6.2434, -1.4927) (-6.2621, -1.5127) (-6.2807, -1.5329) (-6.2991, -1.5533) (-6.3175, -1.5738) (-6.3358, -1.5946) (-6.354, -1.6155) (-6.372, -1.6367) (-6.39, -1.658) (-6.4079, -1.6795) (-6.4256, -1.7012) (-6.4432, -1.7231) (-6.4607, -1.7451) (-6.4781, -1.7674) (-6.4954, -1.7898) (-6.5126, -1.8124) (-6.5297, -1.8352) (-6.5466, -1.8581) (-6.5635, -1.8812) (-6.5802, -1.9045) (-6.5968, -1.928) (-6.6133, -1.9516) (-6.6297, -1.9754) (-6.6459, -1.9994) (-6.6588, -2.0187) (-6.6685, -2.0333) (-6.6749, -2.043) (-6.6781, -2.0479) knots 0 0 0 0 0 0 0.01428571 0.02857143 0.04285714 0.05714286 0.07142857 0.08571429 0.1 0.11428571 0.12857143 0.14285714 0.15714286 0.17142857 0.18571429 0.2 0.21428571 0.22857143 0.24285714 0.25714286 0.27142857 0.28571429 0.3 0.31428571 0.32857143 0.34285714 0.35714286 0.37142857 0.38571429 0.4 0.41428571 0.42857143 0.44285714 0.45714286 0.47142857 0.48571429 0.5 0.51428571 0.52857143 0.54285714 0.55714286 0.57142857 0.58571429 0.6 0.61428571 0.62857143 0.64285714 0.65714286 0.67142857 0.68571429 0.7 0.71428571 0.72857143 0.74285714 0.75714286 0.77142857 0.78571429 0.8 0.81428571 0.82857143 0.84285714 0.85714286 0.87142857 0.88571429 0.9 0.91428571 0.92857143 0.94285714 0.95714286 0.97142857 0.98571429 1 1 1 1 1 1
  arc A22 (-6.6781, -2.0479) -> (-6.432, -2.7238) centre (0, 0) ccw
  spline S11 degree 5 poles (-6.432, -2.7238) (-6.4265, -2.7255) (-6.4153, -2.7288) (-6.3986, -2.7338) (-6.3763, -2.7403) (-6.3484, -2.7482) (-6.3206, -2.7559) (-6.2927, -2.7634) (-6.2649, -2.7707) (-6.2372, -2.7778) (-6.2094, -2.7847) (-6.1817, -2.7914) (-6.1539, -2.7979) (-6.1263, -2.8041) (-6.0986, -2.8102) (-6.071, -2.816) (-6.0434, -2.8217) (-6.0158, -2.8271) (-5.9883, -2.8323) (-5.9608, -2.8373) (-5.9333, -2.8421) (-5.9059, -2.8467) (-5.8785, -2.8511) (-5.8511, -2.8552) (-5.8238, -2.8591) (-5.7966, -2.8629) (-5.7694, -2.8664) (-5.7422, -2.8696) (-5.7151, -2.8727) (-5.688, -2.8755) (-5.661, -2.8782) (-5.6341, -2.8806) (-5.6072, -2.8827) (-5.5803, -2.8847) (-5.5535, -2.8864) (-5.5268, -2.8879) (-5.5002, -2.8892) (-5.4736, -2.8902) (-5.4471, -2.891) (-5.4206, -2.8916) (-5.3942, -2.8919) (-5.3679, -2.892) (-5.3417, -2.8919) (-5.3156, -2.8915) (-5.2895, -2.8908) (-5.2635, -2.89) (-5.2376, -2.8889) (-5.2118, -2.8875) (-5.1861, -2.8859) (-5.1605, -2.884) (-5.135, -2.8819) (-5.1096, -2.8795) (-5.0843, -2.8768) (-5.0591, -2.8739) (-5.034, -2.8706) (-5.0091, -2.8671) (-4.9842, -2.8633) (-4.9595, -2.8593) (-4.9349, -2.855) (-4.9104, -2.8505) (-4.886, -2.8455) (-4.8619, -2.8402) (-4.838, -2.8345) (-4.8142, -2.8283) (-4.7907, -2.8217) (-4.7673, -2.8149) (-4.744, -2.8078) (-4.7208, -2.8006) (-4.6978, -2.7931) (-4.675, -2.785) (-4.6528, -2.7761) (-4.6354, -2.7681) (-4.6227, -2.7614) (-4.6144, -2.7566) (-4.6103, -2.7542) knots -1 -1 -1 -1 -1 -1 -0.98571429 -0.97142857 -0.95714286 -0.94285714 -0.92857143 -0.91428571 -0.9 -0.88571429 -0.87142857 -0.85714286 -0.84285714 -0.82857143 -0.81428571 -0.8 -0.78571429 -0.77142857 -0.75714286 -0.74285714 -0.72857143 -0.71428571 -0.7 -0.68571429 -0.67142857 -0.65714286 -0.64285714 -0.62857143 -0.61428571 -0.6 -0.58571429 -0.57142857 -0.55714286 -0.54285714 -0.52857143 -0.51428571 -0.5 -0.48571429 -0.47142857 -0.45714286 -0.44285714 -0.42857143 -0.41428571 -0.4 -0.38571429 -0.37142857 -0.35714286 -0.34285714 -0.32857143 -0.31428571 -0.3 -0.28571429 -0.27142857 -0.25714286 -0.24285714 -0.22857143 -0.21428571 -0.2 -0.18571429 -0.17142857 -0.15714286 -0.14285714 -0.12857143 -0.11428571 -0.1 -0.08571429 -0.07142857 -0.05714286 -0.04285714 -0.02857143 -0.01428571 0 0 0 0 0 0
  line L11 (-4.6103, -2.7542) -> (-3.8126, -2.2776)
  arc A23 (-3.5431, -2.3391) -> (-3.8126, -2.2776) centre (-3.71, -2.4493) ccw
  arc A24 (-3.5431, -2.3391) -> (-2.9189, -3.0831) centre (0, 0) ccw
  arc A25 (-2.9051, -3.3592) -> (-2.9189, -3.0831) centre (-3.0564, -3.2283) ccw
  line L12 (-2.9051, -3.3592) -> (-3.5129, -4.062)
  spline S12 degree 5 poles (-3.5129, -4.062) (-3.5161, -4.0656) (-3.5222, -4.073) (-3.531, -4.0843) (-3.5419, -4.1) (-3.5545, -4.1204) (-3.5664, -4.1414) (-3.5778, -4.1628) (-3.589, -4.1843) (-3.5999, -4.206) (-3.6107, -4.2279) (-3.6213, -4.25) (-3.6315, -4.2723) (-3.6413, -4.2948) (-3.6508, -4.3177) (-3.6598, -4.3408) (-3.6686, -4.3641) (-3.6771, -4.3876) (-3.6853, -4.4113) (-3.6933, -4.4351) (-3.7011, -4.4591) (-3.7087, -4.4832) (-3.716, -4.5075) (-3.723, -4.5319) (-3.7298, -4.5565) (-3.7363, -4.5813) (-3.7426, -4.6062) (-3.7487, -4.6312) (-3.7545, -4.6564) (-3.7601, -4.6817) (-3.7654, -4.7072) (-3.7706, -4.7327) (-3.7755, -4.7584) (-3.7802, -4.7842) (-3.7847, -4.8101) (-3.7889, -4.8361) (-3.793, -4.8623) (-3.7968, -4.8885) (-3.8004, -4.9149) (-3.8037, -4.9414) (-3.8069, -4.968) (-3.8099, -4.9946) (-3.8126, -5.0214) (-3.8151, -5.0483) (-3.8175, -5.0752) (-3.8196, -5.1023) (-3.8215, -5.1294) (-3.8232, -5.1567) (-3.8247, -5.184) (-3.8259, -5.2114) (-3.827, -5.2389) (-3.8279, -5.2664) (-3.8285, -5.2941) (-3.829, -5.3218) (-3.8292, -5.3496) (-3.8293, -5.3775) (-3.8291, -5.4055) (-3.8288, -5.4335) (-3.8282, -5.4616) (-3.8275, -5.4897) (-3.8265, -5.518) (-3.8253, -5.5463) (-3.824, -5.5746) (-3.8224, -5.603) (-3.8206, -5.6315) (-3.8187, -5.66) (-3.8165, -5.6886) (-3.8142, -5.7173) (-3.8116, -5.746) (-3.8088, -5.7747) (-3.8059, -5.8036) (-3.8034, -5.8266) (-3.8014, -5.844) (-3.8, -5.8556) (-3.7993, -5.8613) knots 0 0 0 0 0 0 0.01428571 0.02857143 0.04285714 0.05714286 0.07142857 0.08571429 0.1 0.11428571 0.12857143 0.14285714 0.15714286 0.17142857 0.18571429 0.2 0.21428571 0.22857143 0.24285714 0.25714286 0.27142857 0.28571429 0.3 0.31428571 0.32857143 0.34285714 0.35714286 0.37142857 0.38571429 0.4 0.41428571 0.42857143 0.44285714 0.45714286 0.47142857 0.48571429 0.5 0.51428571 0.52857143 0.54285714 0.55714286 0.57142857 0.58571429 0.6 0.61428571 0.62857143 0.64285714 0.65714286 0.67142857 0.68571429 0.7 0.71428571 0.72857143 0.74285714 0.75714286 0.77142857 0.78571429 0.8 0.81428571 0.82857143 0.84285714 0.85714286 0.87142857 0.88571429 0.9 0.91428571 0.92857143 0.94285714 0.95714286 0.97142857 0.98571429 1 1 1 1 1 1
  arc A26 (-3.7993, -5.8613) -> (-3.1764, -6.221) centre (0, 0) ccw
  spline S13 degree 5 poles (-3.1764, -6.221) (-3.171, -6.2187) (-3.1603, -6.2141) (-3.1443, -6.2071) (-3.1231, -6.1978) (-3.0967, -6.1859) (-3.0704, -6.1739) (-3.0442, -6.1618) (-3.0182, -6.1495) (-2.9924, -6.1371) (-2.9667, -6.1245) (-2.9412, -6.1118) (-2.9158, -6.099) (-2.8905, -6.086) (-2.8654, -6.0728) (-2.8405, -6.0595) (-2.8158, -6.0461) (-2.7911, -6.0326) (-2.7667, -6.0189) (-2.7424, -6.005) (-2.7183, -5.991) (-2.6943, -5.9769) (-2.6706, -5.9627) (-2.6469, -5.9483) (-2.6235, -5.9337) (-2.6002, -5.9191) (-2.5771, -5.9042) (-2.5542, -5.8893) (-2.5315, -5.8742) (-2.5089, -5.859) (-2.4865, -5.8436) (-2.4644, -5.8281) (-2.4424, -5.8125) (-2.4205, -5.7968) (-2.3989, -5.7809) (-2.3775, -5.7648) (-2.3563, -5.7487) (-2.3352, -5.7324) (-2.3144, -5.7159) (-2.2938, -5.6994) (-2.2733, -5.6827) (-2.2531, -5.6659) (-2.2331, -5.6489) (-2.2134, -5.6318) (-2.1938, -5.6145) (-2.1745, -5.5972) (-2.1553, -5.5797) (-2.1365, -5.5621) (-2.1178, -5.5443) (-2.0994, -5.5264) (-2.0812, -5.5084) (-2.0632, -5.4902) (-2.0456, -5.4719) (-2.0282, -5.4534) (-2.0111, -5.4348) (-1.9942, -5.4161) (-1.9776, -5.3972) (-1.9613, -5.3783) (-1.9451, -5.3591) (-1.9293, -5.3399) (-1.9138, -5.3205) (-1.8988, -5.3009) (-1.8841, -5.2811) (-1.8699, -5.2611) (-1.8561, -5.2409) (-1.8426, -5.2207) (-1.8292, -5.2003) (-1.8161, -5.1799) (-1.8033, -5.1593) (-1.7911, -5.1385) (-1.7797, -5.1174) (-1.7716, -5.1001) (-1.7662, -5.0868) (-1.7629, -5.0778) (-1.7613, -5.0733) knots -1 -1 -1 -1 -1 -1 -0.98571429 -0.97142857 -0.95714286 -0.94285714 -0.92857143 -0.91428571 -0.9 -0.88571429 -0.87142857 -0.85714286 -0.84285714 -0.82857143 -0.81428571 -0.8 -0.78571429 -0.77142857 -0.75714286 -0.74285714 -0.72857143 -0.71428571 -0.7 -0.68571429 -0.67142857 -0.65714286 -0.64285714 -0.62857143 -0.61428571 -0.6 -0.58571429 -0.57142857 -0.55714286 -0.54285714 -0.52857143 -0.51428571 -0.5 -0.48571429 -0.47142857 -0.45714286 -0.44285714 -0.42857143 -0.41428571 -0.4 -0.38571429 -0.37142857 -0.35714286 -0.34285714 -0.32857143 -0.31428571 -0.3 -0.28571429 -0.27142857 -0.25714286 -0.24285714 -0.22857143 -0.21428571 -0.2 -0.18571429 -0.17142857 -0.15714286 -0.14285714 -0.12857143 -0.11428571 -0.1 -0.08571429 -0.07142857 -0.05714286 -0.04285714 -0.02857143 -0.01428571 0 0 0 0 0 0
  line L13 (-1.7613, -5.0733) -> (-1.4566, -4.1955)
  arc A27 (-1.2106, -4.0694) -> (-1.4566, -4.1955) centre (-1.2676, -4.261) ccw
  arc A28 (-1.2106, -4.0694) -> (-0.2542, -4.238) centre (0, 0) ccw
  arc A29 (-0.0662, -4.4406) -> (-0.2542, -4.238) centre (-0.2662, -4.4376) ccw
  line L14 (-0.0662, -4.4406) -> (-0.08, -5.3697)
  spline S14 degree 5 poles (-0.08, -5.3697) (-0.0801, -5.3745) (-0.0801, -5.3841) (-0.0795, -5.3984) (-0.0778, -5.4175) (-0.0744, -5.4412) (-0.07, -5.4649) (-0.065, -5.4886) (-0.0597, -5.5123) (-0.0541, -5.536) (-0.0483, -5.5597) (-0.0422, -5.5834) (-0.0357, -5.607) (-0.0288, -5.6306) (-0.0213, -5.6542) (-0.0134, -5.6777) (-0.0051, -5.7012) (0.0035, -5.7247) (0.0124, -5.7481) (0.0216, -5.7715) (0.031, -5.7949) (0.0407, -5.8182) (0.0507, -5.8415) (0.0611, -5.8648) (0.0717, -5.888) (0.0826, -5.9111) (0.0938, -5.9343) (0.1053, -5.9573) (0.117, -5.9804) (0.129, -6.0033) (0.1412, -6.0263) (0.1537, -6.0492) (0.1664, -6.072) (0.1794, -6.0948) (0.1926, -6.1175) (0.2061, -6.1402) (0.2198, -6.1628) (0.2338, -6.1854) (0.248, -6.2079) (0.2624, -6.2303) (0.2771, -6.2527) (0.292, -6.275) (0.3071, -6.2973) (0.3224, -6.3195) (0.3379, -6.3417) (0.3537, -6.3638) (0.3697, -6.3858) (0.3859, -6.4077) (0.4023, -6.4296) (0.419, -6.4514) (0.4358, -6.4732) (0.4529, -6.4948) (0.4702, -6.5164) (0.4876, -6.538) (0.5053, -6.5594) (0.5232, -6.5808) (0.5413, -6.6021) (0.5596, -6.6234) (0.578, -6.6445) (0.5967, -6.6656) (0.6156, -6.6866) (0.6347, -6.7076) (0.654, -6.7284) (0.6734, -6.7492) (0.6931, -6.7698) (0.7129, -6.7904) (0.733, -6.811) (0.7532, -6.8314) (0.7736, -6.8517) (0.7942, -6.872) (0.815, -6.8922) (0.8317, -6.9082) (0.8444, -6.9202) (0.8529, -6.9282) (0.8571, -6.9322) knots 0 0 0 0 0 0 0.01428571 0.02857143 0.04285714 0.05714286 0.07142857 0.08571429 0.1 0.11428571 0.12857143 0.14285714 0.15714286 0.17142857 0.18571429 0.2 0.21428571 0.22857143 0.24285714 0.25714286 0.27142857 0.28571429 0.3 0.31428571 0.32857143 0.34285714 0.35714286 0.37142857 0.38571429 0.4 0.41428571 0.42857143 0.44285714 0.45714286 0.47142857 0.48571429 0.5 0.51428571 0.52857143 0.54285714 0.55714286 0.57142857 0.58571429 0.6 0.61428571 0.62857143 0.64285714 0.65714286 0.67142857 0.68571429 0.7 0.71428571 0.72857143 0.74285714 0.75714286 0.77142857 0.78571429 0.8 0.81428571 0.82857143 0.84285714 0.85714286 0.87142857 0.88571429 0.9 0.91428571 0.92857143 0.94285714 0.95714286 0.97142857 0.98571429 1 1 1 1 1 1
  arc A30 (0.8571, -6.9322) -> (1.5655, -6.8073) centre (0, 0) ccw
  spline S15 degree 5 poles (1.5655, -6.8073) (1.5681, -6.8021) (1.5734, -6.7917) (1.5812, -6.7761) (1.5914, -6.7552) (1.6041, -6.7292) (1.6165, -6.7031) (1.6287, -6.677) (1.6407, -6.6509) (1.6525, -6.6248) (1.6641, -6.5986) (1.6755, -6.5725) (1.6867, -6.5463) (1.6977, -6.5201) (1.7085, -6.4939) (1.719, -6.4677) (1.7294, -6.4415) (1.7395, -6.4153) (1.7494, -6.3891) (1.7591, -6.3629) (1.7686, -6.3367) (1.7779, -6.3105) (1.787, -6.2843) (1.7958, -6.2581) (1.8044, -6.2318) (1.8128, -6.2057) (1.821, -6.1795) (1.8289, -6.1533) (1.8366, -6.1271) (1.8441, -6.1009) (1.8514, -6.0748) (1.8585, -6.0487) (1.8653, -6.0226) (1.8718, -5.9965) (1.8782, -5.9704) (1.8843, -5.9443) (1.8902, -5.9183) (1.8958, -5.8923) (1.9012, -5.8663) (1.9064, -5.8404) (1.9113, -5.8145) (1.9159, -5.7886) (1.9204, -5.7627) (1.9245, -5.7369) (1.9284, -5.7111) (1.9321, -5.6854) (1.9355, -5.6597) (1.9386, -5.6341) (1.9415, -5.6085) (1.9441, -5.5829) (1.9464, -5.5574) (1.9485, -5.532) (1.9502, -5.5066) (1.9517, -5.4813) (1.9528, -5.456) (1.9537, -5.4308) (1.9543, -5.4057) (1.9547, -5.3807) (1.9547, -5.3557) (1.9545, -5.3308) (1.9539, -5.3059) (1.9528, -5.2812) (1.9513, -5.2567) (1.9493, -5.2322) (1.947, -5.2079) (1.9443, -5.1836) (1.9414, -5.1595) (1.9383, -5.1354) (1.9349, -5.1114) (1.9309, -5.0876) (1.926, -5.0641) (1.9211, -5.0457) (1.9167, -5.032) (1.9135, -5.023) (1.9118, -5.0185) knots -1 -1 -1 -1 -1 -1 -0.98571429 -0.97142857 -0.95714286 -0.94285714 -0.92857143 -0.91428571 -0.9 -0.88571429 -0.87142857 -0.85714286 -0.84285714 -0.82857143 -0.81428571 -0.8 -0.78571429 -0.77142857 -0.75714286 -0.74285714 -0.72857143 -0.71428571 -0.7 -0.68571429 -0.67142857 -0.65714286 -0.64285714 -0.62857143 -0.61428571 -0.6 -0.58571429 -0.57142857 -0.55714286 -0.54285714 -0.52857143 -0.51428571 -0.5 -0.48571429 -0.47142857 -0.45714286 -0.44285714 -0.42857143 -0.41428571 -0.4 -0.38571429 -0.37142857 -0.35714286 -0.34285714 -0.32857143 -0.31428571 -0.3 -0.28571429 -0.27142857 -0.25714286 -0.24285714 -0.22857143 -0.21428571 -0.2 -0.18571429 -0.17142857 -0.15714286 -0.14285714 -0.12857143 -0.11428571 -0.1 -0.08571429 -0.07142857 -0.05714286 -0.04285714 -0.02857143 -0.01428571 0 0 0 0 0 0
  line L15 (1.9118, -5.0185) -> (1.581, -4.1502)
  arc A31 (1.6883, -3.8955) -> (1.581, -4.1502) centre (1.7679, -4.079) ccw
  arc A32 (1.6883, -3.8955) -> (2.5294, -3.4099) centre (0, 0) ccw
  arc A33 (2.8037, -3.4443) -> (2.5294, -3.4099) centre (2.6486, -3.5705) ccw
  line L16 (2.8037, -3.4443) -> (3.3903, -4.1649)
  spline S16 degree 5 poles (3.3903, -4.1649) (3.3933, -4.1686) (3.3995, -4.1759) (3.4091, -4.1866) (3.4227, -4.2001) (3.4406, -4.216) (3.4592, -4.2314) (3.4782, -4.2463) (3.4975, -4.261) (3.517, -4.2756) (3.5367, -4.2901) (3.5566, -4.3043) (3.5768, -4.3182) (3.5973, -4.3318) (3.6181, -4.3451) (3.6393, -4.358) (3.6608, -4.3707) (3.6825, -4.3831) (3.7043, -4.3953) (3.7264, -4.4074) (3.7486, -4.4192) (3.7711, -4.4309) (3.7937, -4.4423) (3.8166, -4.4534) (3.8396, -4.4644) (3.8629, -4.4751) (3.8863, -4.4856) (3.9099, -4.4959) (3.9337, -4.506) (3.9577, -4.5159) (3.9818, -4.5256) (4.0061, -4.5351) (4.0305, -4.5444) (4.0551, -4.5535) (4.0798, -4.5624) (4.1047, -4.5712) (4.1298, -4.5797) (4.155, -4.588) (4.1803, -4.5961) (4.2058, -4.604) (4.2314, -4.6118) (4.2572, -4.6193) (4.2831, -4.6266) (4.3091, -4.6338) (4.3352, -4.6408) (4.3615, -4.6475) (4.3879, -4.6541) (4.4144, -4.6605) (4.4411, -4.6667) (4.4679, -4.6728) (4.4947, -4.6786) (4.5217, -4.6842) (4.5489, -4.6897) (4.5761, -4.6949) (4.6034, -4.7) (4.6309, -4.7049) (4.6584, -4.7096) (4.6861, -4.7141) (4.7138, -4.7185) (4.7417, -4.7226) (4.7697, -4.7266) (4.7977, -4.7303) (4.8259, -4.7339) (4.8542, -4.7373) (4.8825, -4.7405) (4.9109, -4.7435) (4.9395, -4.7464) (4.9681, -4.749) (4.9968, -4.7515) (5.0256, -4.7538) (5.0545, -4.7558) (5.0777, -4.7574) (5.0951, -4.7584) (5.1067, -4.7591) (5.1125, -4.7594) knots 0 0 0 0 0 0 0.01428571 0.02857143 0.04285714 0.05714286 0.07142857 0.08571429 0.1 0.11428571 0.12857143 0.14285714 0.15714286 0.17142857 0.18571429 0.2 0.21428571 0.22857143 0.24285714 0.25714286 0.27142857 0.28571429 0.3 0.31428571 0.32857143 0.34285714 0.35714286 0.37142857 0.38571429 0.4 0.41428571 0.42857143 0.44285714 0.45714286 0.47142857 0.48571429 0.5 0.51428571 0.52857143 0.54285714 0.55714286 0.57142857 0.58571429 0.6 0.61428571 0.62857143 0.64285714 0.65714286 0.67142857 0.68571429 0.7 0.71428571 0.72857143 0.74285714 0.75714286 0.77142857 0.78571429 0.8 0.81428571 0.82857143 0.84285714 0.85714286 0.87142857 0.88571429 0.9 0.91428571 0.92857143 0.94285714 0.95714286 0.97142857 0.98571429 1 1 1 1 1 1
  arc A34 (5.1125, -4.7594) -> (5.5749, -4.2084) centre (0, 0) ccw
  spline S17 degree 5 poles (5.5749, -4.2084) (5.5736, -4.2027) (5.5709, -4.1914) (5.5668, -4.1744) (5.5613, -4.1519) (5.5542, -4.1238) (5.547, -4.0958) (5.5396, -4.068) (5.532, -4.0402) (5.5242, -4.0126) (5.5163, -3.9851) (5.5082, -3.9578) (5.5, -3.9305) (5.4916, -3.9034) (5.483, -3.8764) (5.4742, -3.8496) (5.4653, -3.8229) (5.4562, -3.7963) (5.447, -3.7698) (5.4376, -3.7435) (5.428, -3.7173) (5.4182, -3.6913) (5.4083, -3.6654) (5.3983, -3.6396) (5.388, -3.614) (5.3776, -3.5886) (5.367, -3.5632) (5.3563, -3.5381) (5.3454, -3.5131) (5.3343, -3.4882) (5.3231, -3.4635) (5.3117, -3.439) (5.3001, -3.4146) (5.2884, -3.3904) (5.2765, -3.3663) (5.2644, -3.3424) (5.2522, -3.3187) (5.2398, -3.2952) (5.2272, -3.2718) (5.2145, -3.2486) (5.2016, -3.2256) (5.1885, -3.2028) (5.1753, -3.1801) (5.1619, -3.1577) (5.1483, -3.1354) (5.1346, -3.1134) (5.1206, -3.0915) (5.1066, -3.0698) (5.0923, -3.0484) (5.0779, -3.0271) (5.0633, -3.0061) (5.0485, -2.9853) (5.0335, -2.9647) (5.0184, -2.9444) (5.003, -2.9243) (4.9875, -2.9044) (4.9718, -2.8848) (4.956, -2.8654) (4.94, -2.8462) (4.9238, -2.8273) (4.9073, -2.8087) (4.8906, -2.7904) (4.8737, -2.7726) (4.8565, -2.7551) (4.839, -2.738) (4.8214, -2.7211) (4.8036, -2.7045) (4.7858, -2.688) (4.7678, -2.6719) (4.7494, -2.6562) (4.7306, -2.6413) (4.7149, -2.6303) (4.7028, -2.6227) (4.6945, -2.6179) (4.6904, -2.6156) knots -1 -1 -1 -1 -1 -1 -0.98571429 -0.97142857 -0.95714286 -0.94285714 -0.92857143 -0.91428571 -0.9 -0.88571429 -0.87142857 -0.85714286 -0.84285714 -0.82857143 -0.81428571 -0.8 -0.78571429 -0.77142857 -0.75714286 -0.74285714 -0.72857143 -0.71428571 -0.7 -0.68571429 -0.67142857 -0.65714286 -0.64285714 -0.62857143 -0.61428571 -0.6 -0.58571429 -0.57142857 -0.55714286 -0.54285714 -0.52857143 -0.51428571 -0.5 -0.48571429 -0.47142857 -0.45714286 -0.44285714 -0.42857143 -0.41428571 -0.4 -0.38571429 -0.37142857 -0.35714286 -0.34285714 -0.32857143 -0.31428571 -0.3 -0.28571429 -0.27142857 -0.25714286 -0.24285714 -0.22857143 -0.21428571 -0.2 -0.18571429 -0.17142857 -0.15714286 -0.14285714 -0.12857143 -0.11428571 -0.1 -0.08571429 -0.07142857 -0.05714286 -0.04285714 -0.02857143 -0.01428571 0 0 0 0 0 0
  line L17 (4.6904, -2.6156) -> (3.8788, -2.163)
  arc A35 (3.7973, -1.8989) -> (3.8788, -2.163) centre (3.9762, -1.9883) ccw
  circle A36 centre (0, 0) radius 2.5
  circle A37 centre (0, 0) radius 4
  circle A38 centre (0, 0) radius 4
  dimension "d11" = 8
  constraint coincident A0.centre A2.centre
  constraint concentric A0 A38
  measures "d11" diameter of A37
extrude "Extrude4" cut sketch "Sketch4" against normal blind 3 contours A37 A38
named bodies: "Spur Gear (9 teeth)"
